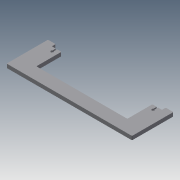
# Autodesk Inventor part: InnerFront
Saved by Autodesk Inventor 2014 (Build 180170000, 170)
## iProperties
Created: 2015-01-19
Part Number: InnerFront
Material: Generic
Document SubType Name: Modeling
Designer: Peele
Density: 1 g/cm^3
Appearance: Default
Author: Peele
Autodesk Inventor part; units mm, degrees
ref_plane "YZ Plane" through (0, 0, 0) normal (1, 0, 0) x (0, 1, 0)
ref_plane "XZ Plane" through (0, 0, 0) normal (0, 1, 0) x (-1, 0, 0)
ref_plane "XY Plane" through (0, 0, 0) normal (0, 0, 1) x (1, 0, 0)
sketch "Sketch1" plane through (0, 0, 0) normal (0, 0, 1) x (1, 0, 0)
  line L0 (100, -30) -> (-100, -30)
  line L1 (-100, -30) -> (-100, 30)
  line L2 (-100, 30) -> (100, 30)
  line L3 (100, 30) -> (100, -30)
  line L4 (100, -30) -> (-100, 30) construction
  line L5 (-100, -30) -> (100, 30) construction
  point P0 (0, 0)
  dimension "d0" = 200
  dimension "d1" = 60
  constraints: 12 end point, 2 midpoint, 2 parallel, 1 horizontal, 1 perpendicular
  measures "d0" distance of L1.end L2.end
  measures "d1" distance of L0.end L1.end
extrude "Extrusion1" add sketch "Sketch1" along normal blind 6
sketch "Sketch2" plane through (0, 0, 6) normal (0, 0, 1) x (1, 0, 0)
  line L0 (-100, -30) -> (100, -30) projected
  line L1 (100, 30) -> (-100, 30) projected
  line L2 (-72.5, -10) -> (72.5, -10)
  line L3 (72.5, -10) -> (72.5, 30)
  line L4 (72.5, 30) -> (-72.5, 30)
  line L5 (-72.5, 30) -> (-72.5, -10)
  line L6 (-72.5, -10) -> (72.5, 30) construction
  line L7 (72.5, -10) -> (-72.5, 30) construction
  point P0 (0, 0)
  point P1 (0, 10)
  dimension "d4" = 145
  dimension "d5" = 20
  constraints: 12 end point, 2 midpoint, 2 parallel, 1 horizontal, 1 perpendicular, 1 point on line, 1 vertical alignment
  measures "d4" distance of L2.start L2.end
  measures "d5" distance between parallel lines of L2 L0
extrude "Extrusion2" cut sketch "Sketch2" against normal through all
sketch "Sketch3" plane through (0, 0, 6) normal (0, 0, 1) x (1, 0, 0)
  line L0 (100, 30) -> (72.5, 30) projected
  line L1 (-100, 30) -> (-87.75, 30)
  line L2 (-87.75, 30) -> (-87.75, 36)
  line L3 (-87.75, 36) -> (-100, 36)
  line L4 (-100, 36) -> (-100, 30)
  line L5 (100, 30) -> (87.75, 30)
  line L6 (87.75, 30) -> (87.75, 36)
  line L7 (87.75, 36) -> (100, 36)
  line L8 (100, 36) -> (100, 30)
  point P0 (0, 0)
  dimension "d9" = 6
  dimension "d20" = 12.25
  constraints: 17 end point, 4 parallel, 2 equal length, 2 horizontal, 2 perpendicular
  measures "d9" distance of L1.end L2.end
  measures "d20" distance of L2.end L3.end
extrude "Extrusion3" add sketch "Sketch3" against normal up to surface (6 mm away)
sketch "Sketch4" plane through (0, 0, 6) normal (0, 0, 1) x (1, 0, 0)
  line L0 (-72.5, 30) -> (-87.75, 30) projected
  line L1 (-81.55, 30) -> (-81.55, 24)
  line L2 (-81.55, 24) -> (-82.55, 24)
  line L3 (-82.55, 24) -> (-82.55, 22.2)
  line L4 (-82.55, 22.2) -> (-81.55, 22.2)
  line L5 (-81.55, 22.2) -> (-81.55, 21)
  line L6 (-81.55, 21) -> (-79.45, 21)
  line L7 (-79.45, 21) -> (-79.45, 22.2)
  line L8 (-79.45, 22.2) -> (-78.45, 22.2)
  line L9 (-78.45, 22.2) -> (-78.45, 24)
  line L10 (-78.45, 24) -> (-79.45, 24)
  line L11 (-79.45, 24) -> (-79.45, 30)
  line L12 (-72.5, -10) -> (-72.5, 30) projected
  line L13 (72.5, -10) -> (-72.5, -10) projected
  line L14 (-80.5, 21) -> (-80.5, 27.2544) construction
  line L15 (-79.45, 30) -> (-81.55, 30)
  point P0 (0, 0)
  point P1 (-80.125, 30)
  dimension "d12" = 2.1
  dimension "d13" = 4.1
  dimension "d15" = 6
  dimension "d16" = 1.8
  dimension "d21" = 8
  dimension "d22" = 9
  constraints: 26 end point, 6 collinear, 6 parallel, 2 equal length, 2 midpoint, 2 perpendicular, 2 point on line, 1 horizontal, 1 vertical
  measures "d12" distance of L5.end L6.end
  measures "d13" distance between parallel lines of L3 L9
  measures "d15" distance of L10.end L11.end
  measures "d16" distance of L8.end L9.end
  measures "d21" distance between parallel lines of L14 L12
  measures "d22" distance between parallel lines of L0 L6
extrude "Extrusion4" cut sketch "Sketch4" against normal blind 10
mirror "Mirror1" about plane through (0, 0, 0) normal (1, 0, 0) of "Extrusion4"
fillet "Fillet1" radius 1 10 edges at (-100, 36, 3) (-87.75, 36, 3) (-72.5, 30, 3) (72.5, 30, 3) (87.75, 36, 3) (100, 36, 3) (100, -30, 3) (72.5, -10, 3) (-72.5, -10, 3) (-100, -30, 3)
body "Solid1"
